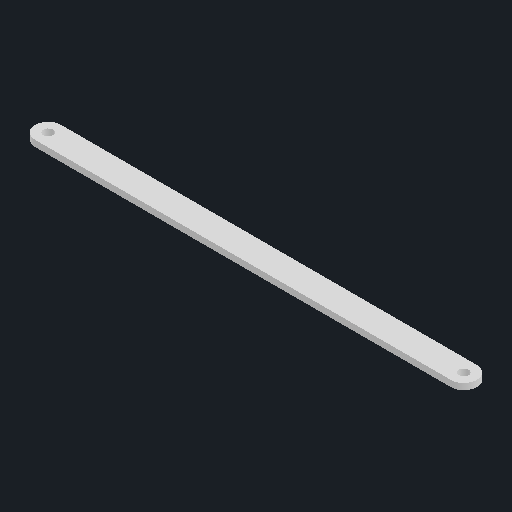
# Autodesk Inventor part: undersideStrip
Saved by Autodesk Inventor 2024.2 (Build 282272000, 272)
## iProperties
Created: 2024-01-29
Part Number: undersideStrip
Material: Generic
Document SubType Name: Sheet Metal
Designer: reima
Density: 1 g/cm^3
Sheet Metal Rule: Default
Appearance: Default
Author: reima
Autodesk Inventor part; units mm, degrees
ref_plane "YZ Plane" through (0, 0, 0) normal (1, 0, 0) x (0, 1, 0)
ref_plane "XZ Plane" through (0, 0, 0) normal (0, 1, 0) x (-1, 0, 0)
ref_plane "XY Plane" through (0, 0, 0) normal (0, 0, 1) x (1, 0, 0)
sketch "Sketch1" plane through (0, 0, 0) normal (0, 1, 0) x (-1, 0, 0)
  circle A0 centre (102.6747, -1.4203) radius 2.1844 construction
  circle A1 centre (-100.5253, -1.4203) radius 2.1844 construction
  circle A2 centre (102.6747, -1.4203) radius 2.3495
  circle A3 centre (-100.5253, -1.4203) radius 2.3495
  circle A4 centre (102.6747, -1.4203) radius 6.35
  circle A5 centre (-100.5253, -1.4203) radius 6.35
  line L0 (102.6747, -7.7703) -> (-100.5253, -7.7703)
  line L1 (102.6747, 4.9297) -> (-100.5253, 4.9297)
  point P0 (0, 0)
  dimension "d0" = 4.699
  dimension "d1" = 4.699
  dimension "d2" = 12.7
  dimension "d3" = 12.7
  measures "d0" diameter of A2
  measures "d1" diameter of A3
  measures "d2" diameter of A4
  measures "d3" diameter of A5
extrude "Plate1" add sketch "Sketch1" along normal blind 3.048
equation "\"d4\" = Thickness"
equation "\"BendRadius\" = Thickness"
equation "\"BendReliefWidth\" = Thickness"
equation "\"BendReliefDepth\" = 0.5 * Thickness"
equation "\"CornerReliefSize\" = 4 * Thickness"
equation "\"MinimumRemnant\" = 2 * Thickness"
equation "\"TransitionRadius\" = BendRadius"
equation "\"JacobiRadiusSize\" = BendRadius"
equation "\"GapSize\" = Thickness"
equation "\"Thickness\" = 3.048"
body "Solid1"
